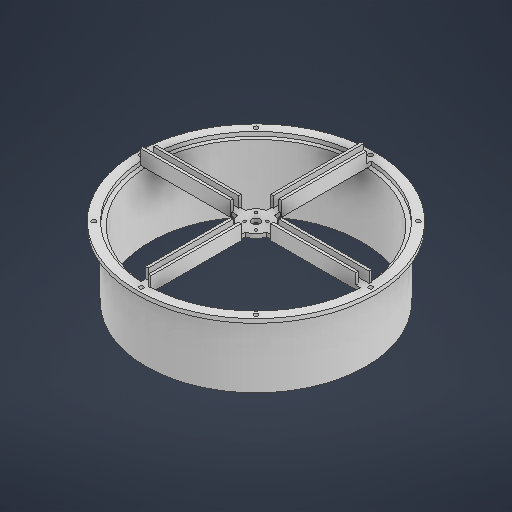
# Autodesk Inventor part: rama-silnik-dol-2
Saved by Autodesk Inventor 2026.2 (Build 302298010, 298A)
## iProperties
Created: 2026-04-17
Part Number: rama-silnik-dol-2
Material: Ogólny
Document SubType Name: Modeling
Designer: macie
Density: 1 g/cm^3
Appearance: Domyślna
Author: macie
Autodesk Inventor part; units mm, degrees
ref_plane "YZ Plane" through (0, 0, 0) normal (1, 0, 0) x (0, 1, 0)
ref_plane "XZ Plane" through (0, 0, 0) normal (0, 1, 0) x (-1, 0, 0)
ref_plane "XY Plane" through (0, 0, 0) normal (0, 0, 1) x (1, 0, 0)
sketch "Szkic1" plane through (0, 0, 0) normal (0, 1, 0) x (-1, 0, 0)
  circle A0 centre (0, 0) radius 11.5
  circle A1 centre (0, 0) radius 3
  line L0 (6, 8) -> (-6, 8)
  line L1 (-6, 8) -> (-6, -8)
  line L2 (-6, -8) -> (6, -8)
  line L3 (6, -8) -> (6, 8)
  line L4 (6, 8) -> (-6, -8) construction
  line L5 (-6, 8) -> (6, -8) construction
  line L6 (0, 8) -> (6, 0)
  line L7 (6, 0) -> (0, -8)
  line L8 (0, -8) -> (-6, 0)
  line L9 (-6, 0) -> (0, 8)
  dimension "d0" = 23
  dimension "d1" = 6
  dimension "d2" = 16
  dimension "d3" = 12
  constraints: 20 end point, 6 midpoint, 3 parallel, 2 centre point, 2 coincident, 1 horizontal, 1 perpendicular
  measures "d0" diameter of A0
  measures "d1" diameter of A1
  measures "d2" distance between parallel lines of L0 L2
  measures "d3" distance between parallel lines of L3 L1
extrude "Wyciągnięcie proste1" add sketch "Szkic1" along normal blind 3 contours A0 | L3 L6 L0 | L9 L1 L0 | L6 L7 L8 L9 | L3 L2 L7 | L8 L2 L1
sketch "Szkic2" plane through (0, 0, 0) normal (0, -1, 0) x (1, 0, 0)
  circle A0 centre (0, 0) radius 11.5 projected
  line L0 (-11.5, 0) -> (-11.5, -3)
  line L1 (-11.5, -3) -> (-82.2, -3)
  line L2 (-82.2, -3) -> (-82.2, 3)
  line L3 (-82.2, 3) -> (-11.5, 3)
  line L4 (-11.5, 3) -> (-11.5, -3)
  line L5 (-11.5, 3) -> (-11.1018, 3)
  line L6 (-11.5, -3) -> (-11.1018, -3)
  circle A1 centre (0, 0) radius 3 projected
  line L7 (3, -11.5) -> (3, -82.2)
  line L8 (-3, -82.2) -> (-3, -11.5)
  line L9 (3, -11.5) -> (3, -11.1018)
  line L10 (0, -11.5) -> (3, -11.5)
  line L11 (-3, -11.5) -> (-3, -11.1018)
  line L12 (-3, -11.5) -> (3, -11.5)
  line L13 (3, -82.2) -> (-3, -82.2)
  line L14 (11.5, 3) -> (82.2, 3)
  line L15 (82.2, -3) -> (11.5, -3)
  line L16 (11.5, 3) -> (11.1018, 3)
  line L17 (11.5, 0) -> (11.5, 3)
  line L18 (11.5, -3) -> (11.1018, -3)
  line L19 (11.5, -3) -> (11.5, 3)
  line L20 (82.2, 3) -> (82.2, -3)
  line L21 (-3, 11.5) -> (-3, 82.2)
  line L22 (3, 82.2) -> (3, 11.5)
  line L23 (-3, 11.5) -> (-3, 11.1018)
  line L24 (0, 11.5) -> (-3, 11.5)
  line L25 (3, 11.5) -> (3, 11.1018)
  line L26 (3, 11.5) -> (-3, 11.5)
  line L27 (-3, 82.2) -> (3, 82.2)
  circle A2 centre (0, 0) radius 82.2547
  circle A3 centre (0, 0) radius 89.2547
  point P0 (-11.5, 0)
  point P1 (0, -11.5)
  point P2 (11.5, 0)
  point P3 (0, 11.5)
  point P4 (11.5, 0)
  point P5 (11.5, 0)
  point P6 (11.5, 0)
  dimension "d15" = 70.7
  dimension "d17" = 6
  dimension "d18" = 3
  dimension "d21" = 360
  dimension "d23" = 7
  constraints: 56 end point, 3 parallel, 3 point on circle, 2 coincident, 2 horizontal, 1 centre point, 1 midpoint, 1 perpendicular, 1 tangent, 1 vertical, 64 other
  measures "d15" distance between parallel lines of L2 L4
  measures "d17" distance between parallel lines of L3 L1
  measures "d18" distance from line of L0.start L3
extrude "Wyciągnięcie proste2" add sketch "Szkic2" against normal blind 3 contours L19 L18 A0 | A0 L16 L17 | L17 L14 L20 L15 L19 | A0 L26 L25 | L9 L10 A0 | A2 L20 | A0 L23 L24 | L24 L21 L27 L22 L26 | L12 L11 A0 | L10 L7 L13 L8 L12 | L27 A2 | A2 L13 | A0 L4 L5 | L6 L0 A0 | L3 L4 L0 L1 L2 | L2 A2 | A3
sketch "Szkic3" plane through (0, 3, 0) normal (0, 1, 0) x (1, 0, 0)
  line L0 (82.2, 3) -> (11.1018, 3) projected
  circle A0 centre (0, 0) radius 89.2547 projected
  line L1 (0, 89.2547) -> (89.2547, 89.2547)
  line L2 (89.2547, 89.2547) -> (89.2547, 0)
  line L3 (89.2547, 0) -> (0, 0)
  line L4 (0, 0) -> (0, 89.2547)
  circle A1 centre (0, 0) radius 3 projected
  line L5 (0, 0) -> (89.2547, 89.2547)
  circle A2 centre (60.6377, 60.6377) radius 3.5
  arc A3 (82.2, 3) -> (3, 82.2) centre (0, 0) ccw projected
  circle A4 centre (0, 85.7547) radius 3.5
  circle A5 centre (-60.6377, 60.6377) radius 3.5
  circle A6 centre (-85.7547, 0) radius 3.5
  circle A7 centre (-60.6377, -60.6377) radius 3.5
  circle A8 centre (0, -85.7547) radius 3.5
  circle A9 centre (60.6377, -60.6377) radius 3.5
  circle A10 centre (85.7547, 0) radius 3.5
  dimension "d42" = 360
  constraints: 10 end point, 8 centre point, 2 parallel, 2 point on circle, 2 tangent, 1 horizontal, 1 perpendicular, 1 point on line, 17 other
hole "Otwór3" at (60.6377, 3, -60.6377) at (0, 3, -85.7547) at (-60.6377, 3, -60.6377) at (-85.7547, 3, 0) at (85.7547, 3, 0) at (-60.6377, 3, 60.6377) at (0, 3, 85.7547) at (60.6377, 3, 60.6377) direction (0, -1, 0) diameter 3.2 end through all
sketch "Szkic5" plane through (0, 3, 0) normal (0, 1, 0) x (1, 0, 0)
  line L0 (9.8995, -1.4142) -> (1.4142, -9.8995)
  line L1 (1.4142, -9.8995) -> (-9.8995, 1.4142)
  line L2 (-9.8995, 1.4142) -> (-1.4142, 9.8995)
  line L3 (-1.4142, 9.8995) -> (9.8995, -1.4142)
  arc A0 (3, -11.1018) -> (11.1018, -3) centre (0, 0) ccw projected
  arc A1 (-11.1018, -3) -> (-3, -11.1018) centre (0, 0) ccw projected
  line L4 (3, -11.1018) -> (-3, -11.1018)
  line L5 (5.6569, -5.6569) -> (4.2426, 4.2426)
  line L6 (4.2426, 4.2426) -> (-5.6569, 5.6569)
  line L7 (-5.6569, 5.6569) -> (-4.2426, -4.2426)
  line L8 (-4.2426, -4.2426) -> (5.6569, -5.6569)
  dimension "d57" = 45
  dimension "d58" = 12
  dimension "d59" = 16
  dimension "d60" = 6
  dimension "d61" = 8
  constraints: 18 end point, 4 midpoint, 3 parallel, 1 horizontal, 1 perpendicular
  measures "d57" angle of L4 L3
  measures "d58" distance between parallel lines of L1 L3
  measures "d59" distance between parallel lines of L2 L0
  measures "d60" distance from line of L3 point (0, 0)
  measures "d61" distance from line of point (0, 0) L0
hole "Otwór4" at (5.6569, 3, 5.6569) at (4.2426, 3, -4.2426) at (-5.6569, 3, -5.6569) at (-4.2426, 3, 4.2426) direction (0, -1, 0) diameter 2.1 end through all
sketch "Szkic6" plane through (0, 3, 0) normal (0, 1, 0) x (1, 0, 0)
  line L0 (-15.1018, 2) -> (-15.1018, 4)
  line L1 (-15.1018, 4) -> (-82.6018, 4)
  line L2 (-82.6018, 4) -> (-82.6018, 2)
  line L3 (-82.6018, 2) -> (-15.1018, 2)
  line L4 (-11.1018, 3) -> (-82.2, 3) projected
  line L5 (-4, -15.1018) -> (-4, -82.6018)
  line L6 (-2, -82.6018) -> (-2, -15.1018)
  line L7 (-4, -82.6018) -> (-2, -82.6018)
  line L8 (-2, -15.1018) -> (-4, -15.1018)
  line L9 (15.1018, -4) -> (82.6018, -4)
  line L10 (82.6018, -2) -> (15.1018, -2)
  line L11 (82.6018, -4) -> (82.6018, -2)
  line L12 (15.1018, -2) -> (15.1018, -4)
  line L13 (4, 15.1018) -> (4, 82.6018)
  line L14 (2, 82.6018) -> (2, 15.1018)
  line L15 (4, 82.6018) -> (2, 82.6018)
  line L16 (2, 15.1018) -> (4, 15.1018)
  line L17 (-82.6018, -2) -> (-82.6018, -4)
  line L18 (-82.6018, -4) -> (-15.1018, -4)
  line L19 (-15.1018, -4) -> (-15.1018, -2)
  line L20 (-15.1018, -2) -> (-82.6018, -2)
  line L21 (-82.2, -3) -> (-11.1018, -3) projected
  line L22 (4, -82.6018) -> (4, -15.1018)
  line L23 (2, -15.1018) -> (2, -82.6018)
  line L24 (2, -82.6018) -> (4, -82.6018)
  line L25 (4, -15.1018) -> (2, -15.1018)
  line L26 (82.6018, 4) -> (15.1018, 4)
  line L27 (15.1018, 2) -> (82.6018, 2)
  line L28 (82.6018, 2) -> (82.6018, 4)
  line L29 (15.1018, 4) -> (15.1018, 2)
  line L30 (-4, 82.6018) -> (-4, 15.1018)
  line L31 (-2, 15.1018) -> (-2, 82.6018)
  line L32 (-2, 82.6018) -> (-4, 82.6018)
  line L33 (-4, 15.1018) -> (-2, 15.1018)
  point P0 (0, 0)
  point P1 (-3, -82.2)
  point P2 (82.2, -3)
  point P3 (3, 82.2)
  dimension "d69" = 2
  dimension "d70" = 1
  dimension "d71" = 4
  dimension "d72" = 67.5
  dimension "d75" = 360
  dimension "d77" = 1
  dimension "d78" = 2
  dimension "d79" = 67.5
  dimension "d80" = 4
  dimension "d83" = 360
  constraints: 56 end point, 3 parallel, 3 perpendicular, 2 vertical, 82 other
  measures "d69" distance between parallel lines of L3 L1
  measures "d70" distance between parallel lines of L3 L4
  measures "d71" distance from line of L4.start L0
  measures "d77" distance between parallel lines of L21 L20
  measures "d78" distance between parallel lines of L18 L20
  measures "d79" distance between parallel lines of L19 L17
  measures "d80" distance from line of L21.end L19
extrude "Wyciągnięcie proste4" add sketch "Szkic6" along normal blind 8 and the other way blind 3
sketch "Szkic7" plane through (-4, 0, 15.1018) normal (-1, 0, 0) x (0, 0, 1)
  line L0 (0, 11) -> (67.5, 11) projected
  line L1 (74.1529, 3) -> (-104.3565, 3) projected
  line L2 (67.5, 11) -> (63.5, 11)
  line L3 (63.5, 11) -> (63.5, 3)
  line L4 (63.5, 3) -> (67.5, 3)
  line L5 (67.5, 3) -> (67.5, 11)
  point P0 (-15.1018, 0)
  dimension "d89" = 4
  constraints: 8 end point, 2 parallel, 1 horizontal, 1 perpendicular, 1 point on line
  measures "d89" distance between parallel lines of L5 L3
extrude "Wyciągnięcie proste5" cut sketch "Szkic7" against normal blind 2
pattern_circular "Szyk kołowy1" count 4 over 360 about axis through (0, 0, 0) along (0, 1, 0) of "Wyciągnięcie proste5"
sketch "Szkic8" plane through (0, 0, 0) normal (0, -1, 0) x (1, 0, 0)
  circle A0 centre (0, 0) radius 79.2547
  circle A1 centre (0, 0) radius 3 projected
  circle A2 centre (0, 0) radius 82.2547
  dimension "d95" = 164.5094
  dimension "d96" = 158.5094
  constraints: 2 centre point, 2 coincident
  measures "d95" diameter of A2
  measures "d96" diameter of A0
extrude "Wyciągnięcie proste6" add sketch "Szkic8" along normal blind 50 contours A2
sketch "Szkic9" plane through (0, 3, 0) normal (0, 1, 0) x (1, 0, 0)
  circle A0 centre (0, 0) radius 3 projected
  circle A1 centre (0, 0) radius 79.2547 projected
  circle A2 centre (0, 0) radius 82.2547
  circle A3 centre (0, 0) radius 79.2547
  line L0 (-4, -82.1574) -> (-4, -79.1537) projected
  line L1 (-4, -82.1574) -> (-4, -79.1537)
  line L2 (-82.1574, 4) -> (-78.6018, 4) projected
  line L3 (-82.1574, 4) -> (-78.6018, 4)
  line L4 (-78.6018, 4) -> (-79.1537, 4)
  line L5 (4, 79.1537) -> (4, 15.1018) projected
  line L6 (4, 79.1537) -> (4, 82.1574)
  line L7 (79.1537, -4) -> (-82.1574, -4)
  line L8 (78.6018, -4) -> (78.6018, -2) projected
  arc A4 (-82.1574, -4) -> (-4, -82.1574) centre (0, 0) ccw projected
  line L9 (-6.4282, -82.0032) -> (-6.3234, -79.0015)
  point P0 (-6.3344, -79.0012)
  dimension "d100" = 3
  dimension "d101" = 2
  constraints: 12 end point, 6 point on circle, 3 collinear, 2 centre point, 2 coincident, 1 concentric, 1 perpendicular, 1 point on line
  measures "d100" radial gap between concentric circles of A2 A1
  measures "d101" angle of L0 L9
equation "\"d77\" = d70"
equation "\"d78\" = d69"
equation "\"d79\" = d72"
equation "\"d80\" = d71"
